Autodesk Fusion 360 part; units mm, degrees
(part 3 of 5)
  line L3 (45.4352, 19.4331, 2.5409) -> (44.7866, 20.9539, 2.7513) construction
  line L4 (44.7866, 20.9539, 2.7513) -> (44.0616, 22.4421, 2.9616) construction
  line L5 (44.0616, 22.4421, 2.9616) -> (43.2623, 23.8896, 3.172) construction
  line L6 (43.2623, 23.8896, 3.172) -> (39.2446, 31.1652, 4.2293) construction
  line L7 (39.2446, 31.1652, 4.2293) -> (33.358, 37.3986, 5.2866) construction
  line L8 (33.358, 37.3986, 5.2866) -> (26.324, 41.8256, 6.3439) construction
  line L9 (26.324, 41.8256, 6.3439) -> (19.2902, 46.2525, 7.4011) construction
  line L10 (19.2902, 46.2525, 7.4011) -> (11.1241, 48.8637, 8.4584) construction
  line L11 (11.1241, 48.8637, 8.4584) -> (2.8268, 49.3391, 9.5157) construction
  line L12 (2.8268, 49.3391, 9.5157) -> (-5.4704, 49.8145, 10.5729) construction
  line L13 (-5.4704, 49.8145, 10.5729) -> (-13.8811, 48.1531, 11.6302) construction
  line L14 (-13.8811, 48.1531, 11.6302) -> (-21.3743, 44.5587, 12.6874) construction
  line L15 (-21.3743, 44.5587, 12.6874) -> (-28.8674, 40.9643, 13.7447) construction
  line L16 (-28.8674, 40.9643, 13.7447) -> (-35.4271, 35.4447, 14.8019) construction
  line L17 (-35.4271, 35.4447, 14.8019) -> (-40.2493, 28.6763, 15.8591) construction
  line L18 (-40.2493, 28.6763, 15.8591) -> (-45.0715, 21.908, 16.9163) construction
  line L19 (-45.0715, 21.908, 16.9163) -> (-48.146, 13.9055, 17.9735) construction
  line L20 (-48.146, 13.9055, 17.9735) -> (-49.096, 5.6496, 19.0307) construction
  line L21 (-49.096, 5.6496, 19.0307) -> (-50.046, -2.606, 20.0879) construction
  line L22 (-50.046, -2.606, 20.0879) -> (-48.8696, -11.0975, 21.1451) construction
  line L23 (-48.8696, -11.0975, 21.1451) -> (-45.711, -18.784, 22.2022) construction
  line L24 (-45.711, -18.784, 22.2022) -> (-42.5525, -26.4703, 23.2594) construction
  line L25 (-42.5525, -26.4703, 23.2594) -> (-37.4186, -33.3353, 24.3165) construction
  line L26 (-37.4186, -33.3353, 24.3165) -> (-30.9385, -38.5376, 25.3737) construction
  line L27 (-30.9385, -38.5376, 25.3737) -> (-24.4586, -43.7398, 26.4308) construction
  line L28 (-24.4586, -43.7398, 26.4308) -> (-16.6463, -47.2683, 27.4879) construction
  line L29 (-16.6463, -47.2683, 27.4879) -> (-8.4592, -48.6906, 28.545) construction
  line L30 (-8.4592, -48.6906, 28.545) -> (-0.2722, -50.113, 29.6021) construction
  line L31 (-0.2722, -50.113, 29.6021) -> (8.2721, -49.4263, 30.6592) construction
  line L32 (8.2721, -49.4263, 30.6592) -> (16.1268, -46.7147, 31.7163) construction
  line L33 (16.1268, -46.7147, 31.7163) -> (23.9813, -44.0032, 32.7734) construction
  line L34 (23.9813, -44.0032, 32.7734) -> (31.1295, -39.2726, 33.8305) construction
  line L35 (31.1295, -39.2726, 33.8305) -> (36.6953, -33.1027, 34.8876) construction
  line L36 (36.6953, -33.1027, 34.8876) -> (42.261, -26.933, 35.9446) construction
  line L37 (42.261, -26.933, 35.9446) -> (46.2326, -19.3372, 37.0017) construction
  line L38 (46.2326, -19.3372, 37.0017) -> (48.1234, -11.246, 38.0587) construction
  line L39 (48.1234, -11.246, 38.0587) -> (50.0142, -3.155, 39.1157) construction
  line L40 (50.0142, -3.155, 39.1157) -> (49.8203, 5.4141, 40.1728) construction
  line L41 (49.8203, 5.4141, 40.1728) -> (47.5655, 13.4113, 41.2298) construction
  line L42 (47.5655, 13.4113, 41.2298) -> (45.3107, 21.4083, 42.2868) construction
  line L43 (45.3107, 21.4083, 42.2868) -> (40.9999, 28.8164, 43.3438) construction
  line L44 (40.9999, 28.8164, 43.3438) -> (35.1612, 34.7279, 44.4008) construction
  line L45 (35.1612, 34.7279, 44.4008) -> (29.3227, 40.6393, 45.4577) construction
  line L46 (29.3227, 40.6393, 45.4577) -> (21.9688, 45.0415, 46.5147) construction
  line L47 (21.9688, 45.0415, 46.5147) -> (14.0006, 47.3954, 47.5717) construction
  line L48 (14.0006, 47.3954, 47.5717) -> (6.0326, 49.7491, 48.6286) construction
  line L49 (6.0326, 49.7491, 48.6286) -> (-2.5328, 50.0495, 49.6856) construction
  line L50 (-2.5328, 50.0495, 49.6856) -> (-10.6461, 48.2597, 50.7425) construction
  line L51 (-10.6461, 48.2597, 50.7425) -> (-18.7593, 46.4699, 51.7995) construction
  line L52 (-18.7593, 46.4699, 51.7995) -> (-26.4031, 42.5939, 52.8564) construction
  line L53 (-26.4031, 42.5939, 52.8564) -> (-32.6413, 37.1064, 53.9133) construction
  line L54 (-32.6413, 37.1064, 53.9133) -> (-38.8792, 31.6191, 54.9702) construction
  line L55 (-38.8792, 31.6191, 54.9702) -> (-43.6983, 24.5321, 56.0271) construction
  line L56 (-43.6983, 24.5321, 56.0271) -> (-46.508, 16.7136, 57.084) construction
  line L57 (-46.508, 16.7136, 57.084) -> (-49.3176, 8.8953, 58.1409) construction
  line L58 (-49.3176, 8.8953, 58.1409) -> (-50.1121, 0.3622, 59.1978) construction
  line L59 (-50.1121, 0.3622, 59.1978) -> (-48.7941, -7.8404, 60.2546) construction
  line L60 (-48.7941, -7.8404, 60.2546) -> (-47.4761, -16.0429, 61.3115) construction
  line L61 (-47.4761, -16.0429, 61.3115) -> (-44.0485, -23.8973, 62.3684) construction
  line L62 (-44.0485, -23.8973, 62.3684) -> (-38.9312, -30.4418, 63.4252) construction
  line L63 (-38.9312, -30.4418, 63.4252) -> (-33.8139, -36.986, 64.482) construction
  line L64 (-33.8139, -36.986, 64.482) -> (-27.0179, -42.2064, 65.5389) construction
  line L65 (-27.0179, -42.2064, 65.5389) -> (-19.3756, -45.4634, 66.5957) construction
  line L66 (-19.3756, -45.4634, 66.5957) -> (-11.7334, -48.7204, 67.6525) construction
  line L67 (-11.7334, -48.7204, 67.6525) -> (-3.2612, -50.0071, 68.7093) construction
  line L68 (-3.2612, -50.0071, 68.7093) -> (5.0034, -49.1661, 69.7661) construction
  line L69 (5.0034, -49.1661, 69.7661) -> (13.2677, -48.3251, 70.8229) construction
  line L70 (13.2677, -48.3251, 70.8229) -> (21.3069, -45.3581, 71.8796) construction
  line L71 (21.3069, -45.3581, 71.8796) -> (28.1362, -40.6287, 72.9364) construction
  line L72 (28.1362, -40.6287, 72.9364) -> (34.9654, -35.8993, 73.9932) construction
  line L73 (34.9654, -35.8993, 73.9932) -> (40.5702, -29.4176, 75.0499) construction
  line L74 (40.5702, -29.4176, 75.0499) -> (44.2643, -21.9774, 76.1067) construction
  line L75 (44.2643, -21.9774, 76.1067) -> (47.9584, -14.5373, 77.1634) construction
  line L76 (47.9584, -14.5373, 77.1634) -> (49.7339, -6.1545, 78.2202) construction
  line L77 (49.7339, -6.1545, 78.2202) -> (49.3735, 2.1444, 79.2769) construction
  line L78 (49.3735, 2.1444, 79.2769) -> (49.013, 10.4431, 80.3336) construction
  line L79 (49.013, 10.4431, 80.3336) -> (46.5175, 18.6401, 81.3903) construction
  line L80 (46.5175, 18.6401, 81.3903) -> (42.1925, 25.7318, 82.447) construction
  line L81 (42.1925, 25.7318, 82.447) -> (37.8676, 32.8234, 83.5037) construction
  line L82 (37.8676, 32.8234, 83.5037) -> (31.7225, 38.7945, 84.5604) construction
  line L83 (31.7225, 38.7945, 84.5604) -> (24.5097, 42.914, 85.617) construction
  line L84 (24.5097, 42.914, 85.617) -> (17.2971, 47.0334, 86.6737) construction
  line L85 (17.2971, 47.0334, 86.6737) -> (9.0322, 49.2925, 87.7304) construction
  line L86 (9.0322, 49.2925, 87.7304) -> (0.7269, 49.4147, 88.787) construction
  line L87 (0.7269, 49.4147, 88.787) -> (-7.5781, 49.5368, 89.8437) construction
  line L88 (-7.5781, 49.5368, 89.8437) -> (-15.9057, 47.5219, 90.9003) construction
  line L89 (-15.9057, 47.5219, 90.9003) -> (-23.2363, 43.6166, 91.9569) construction
  line L90 (-23.2363, 43.6166, 91.9569) -> (-30.5667, 39.7114, 93.0135) construction
  line L91 (-30.5667, 39.7114, 93.0135) -> (-36.8845, 33.9243, 94.0701) construction
  line L92 (-36.8845, 33.9243, 94.0701) -> (-41.4161, 26.9637, 95.1268) construction
  line L93 (-41.4161, 26.9637, 95.1268) -> (-45.9477, 20.0033, 96.1833) construction
  line L94 (-45.9477, 20.0033, 96.1833) -> (-48.6835, 11.8843, 97.2399) construction
  line L95 (-48.6835, 11.8843, 97.2399) -> (-49.2886, 3.6009, 98.2965) construction
  line L96 (-49.2886, 3.6009, 98.2965) -> (-49.8938, -4.6824, 99.3531) construction
  line L97 (-49.8938, -4.6824, 99.3531) -> (-48.3671, -13.1126, 100.4096) construction
  line L98 (-48.3671, -13.1126, 100.4096) -> (-44.8954, -20.6576, 101.4662) construction
  line L99 (-44.8954, -20.6576, 101.4662) -> (-41.4239, -28.2024, 102.5227) construction
  line L100 (-41.4239, -28.2024, 102.5227) -> (-36.0148, -34.846, 103.5793) construction
  line L101 (-36.0148, -34.846, 103.5793) -> (-29.3305, -39.7751, 104.6358) construction
  line L102 (-29.3305, -39.7751, 104.6358) -> (-22.6463, -44.7041, 105.6923) construction
  line L103 (-22.6463, -44.7041, 105.6923) -> (-14.7012, -47.9081, 106.7488) construction
  line L104 (-14.7012, -47.9081, 106.7488) -> (-6.4676, -48.995, 107.8054) construction
  line L105 (-6.4676, -48.995, 107.8054) -> (1.7658, -50.0818, 108.8619) construction
  line L106 (1.7658, -50.0818, 108.8619) -> (10.27, -49.0493, 109.9183) construction
  line L107 (10.27, -49.0493, 109.9183) -> (18.0041, -46.0238, 110.9748) construction
  line L108 (18.0041, -46.0238, 110.9748) -> (25.738, -42.9983, 112.0313) construction
  line L109 (25.738, -42.9983, 112.0313) -> (32.6854, -37.9864, 113.0878) construction
  line L110 (32.6854, -37.9864, 113.0878) -> (37.9957, -31.6016, 114.1442) construction
  line L111 (37.9957, -31.6016, 114.1442) -> (43.306, -25.2168, 115.2007) construction
  line L112 (43.306, -25.2168, 115.2007) -> (46.9681, -17.4728, 116.2571) construction
  line L113 (46.9681, -17.4728, 116.2571) -> (48.5337, -9.3173, 117.3136) construction
  line L114 (48.5337, -9.3173, 117.3136) -> (50.0994, -1.1619, 118.37) construction
  line L115 (50.0994, -1.1619, 118.37) -> (49.5653, 7.3875, 119.4264) construction
  line L116 (49.5653, 7.3875, 119.4264) -> (46.997, 15.2846, 120.4828) construction
  line L117 (46.997, 15.2846, 120.4828) -> (44.4287, 23.1815, 121.5392) construction
  line L118 (44.4287, 23.1815, 121.5392) -> (39.8317, 30.4094, 122.5956) construction
  line L119 (39.8317, 30.4094, 122.5956) -> (33.7686, 36.0835, 123.652) construction
  line L120 (33.7686, 36.0835, 123.652) -> (27.7056, 41.7575, 124.7084) construction
  line L121 (27.7056, 41.7575, 124.7084) -> (20.1894, 45.8659, 125.7648) construction
  line L122 (20.1894, 45.8659, 125.7648) -> (12.14, 47.9057, 126.8211) construction
  line L123 (12.14, 47.9057, 126.8211) -> (4.0907, 49.9455, 127.8775) construction
  line L124 (4.0907, 49.9455, 127.8775) -> (-4.4747, 49.9126, 128.9338) construction
  line L125 (-4.4747, 49.9126, 128.9338) -> (-12.508, 47.8109, 129.9902) construction
  line L126 (-12.508, 47.8109, 129.9902) -> (-20.5412, 45.7093, 131.0465) construction
  line L127 (-20.5412, 45.7093, 131.0465) -> (-28.0252, 41.5436, 132.1029) construction
  line L128 (-28.0252, 41.5436, 132.1029) -> (-34.0443, 35.8235, 133.1592) construction
  line L129 (-34.0443, 35.8235, 133.1592) -> (-40.0632, 30.1035, 134.2155) construction
  line L130 (-40.0632, 30.1035, 134.2155) -> (-44.6044, 22.8414, 135.2718) construction
  line L131 (-44.6044, 22.8414, 135.2718) -> (-47.1122, 14.9259, 136.3281) construction
  line L132 (-47.1122, 14.9259, 136.3281) -> (-49.6199, 7.0105, 137.3844) construction
  line L133 (-49.6199, 7.0105, 137.3844) -> (-50.0889, -1.5416, 138.4407) construction
  line L134 (-50.0889, -1.5416, 138.4407) -> (-48.462, -9.6838, 139.4969) construction
  line L135 (-48.462, -9.6838, 139.4969) -> (-46.835, -17.8258, 140.5532) construction
  line L136 (-46.835, -17.8258, 140.5532) -> (-43.1155, -25.5407, 141.6095) construction
  line L137 (-43.1155, -25.5407, 141.6095) -> (-37.7587, -31.8844, 142.6657) construction
  line L138 (-37.7587, -31.8844, 142.6657) -> (-32.402, -38.2281, 143.7219) construction
  line L139 (-32.402, -38.2281, 143.7219) -> (-25.4193, -43.1872, 144.7782) construction
  line L140 (-25.4193, -43.1872, 144.7782) -> (-17.665, -46.155, 145.8344) construction
  line L141 (-17.665, -46.155, 145.8344) -> (-9.911, -49.1227, 146.8906) construction
  line L142 (-9.911, -49.1227, 146.8906) -> (-1.4018, -50.093, 147.9468) construction
  line L143 (-1.4018, -50.093, 147.9468) -> (6.8213, -48.947, 149.0031) construction
  line L144 (6.8213, -48.947, 149.0031) -> (15.0443, -47.801, 150.0592) construction
  line L145 (15.0443, -47.801, 150.0592) -> (22.9638, -44.5413, 151.1154) construction
  line L146 (22.9638, -44.5413, 151.1154) -> (29.6109, -39.5668, 152.1716) construction
  line L147 (29.6109, -39.5668, 152.1716) -> (36.2579, -34.5923, 153.2278) construction
  line L148 (36.2579, -34.5923, 153.2278) -> (41.6184, -27.9136, 154.284) construction
  line L149 (41.6184, -27.9136, 154.284) -> (45.0367, -20.3478, 155.3401) construction
  line L150 (45.0367, -20.3478, 155.3401) -> (48.4549, -12.782, 156.3963) construction
  line L151 (48.4549, -12.782, 156.3963) -> (49.9237, -4.3452, 157.4524) construction
  line L152 (49.9237, -4.3452, 157.4524) -> (49.2634, 3.9305, 158.5085) construction
  line L153 (49.2634, 3.9305, 158.5085) -> (48.6032, 12.2061, 159.5647) construction
  line L154 (48.6032, 12.2061, 159.5647) -> (45.8153, 20.3031, 160.6208) construction
  line L155 (45.8153, 20.3031, 160.6208) -> (41.2409, 27.231, 161.6769) construction
  line L156 (41.2409, 27.231, 161.6769) -> (36.6665, 34.1588, 162.733) construction
  line L157 (36.6665, 34.1588, 162.733) -> (30.3154, 39.9028, 163.7891) construction
  line L158 (30.3154, 39.9028, 163.7891) -> (22.9644, 43.7604, 164.8452) construction
  line L159 (22.9644, 43.7604, 164.8452) -> (15.6136, 47.6179, 165.9013) construction
  line L160 (15.6136, 47.6179, 165.9013) -> (7.2785, 49.581, 166.9574) construction
  line L161 (7.2785, 49.581, 166.9574) -> (-1.0213, 49.4094, 168.0134) construction
  line L162 (-1.0213, 49.4094, 168.0134) -> (-9.3208, 49.2379, 169.0695) construction
  line L163 (-9.3208, 49.2379, 169.0695) -> (-17.5675, 46.9322, 170.1255) construction
  line L164 (-17.5675, 46.9322, 170.1255) -> (-24.7525, 42.7744, 171.1816) construction
  line L165 (-24.7525, 42.7744, 171.1816) -> (-31.9374, 38.6166, 172.2376) construction
  line L166 (-31.9374, 38.6166, 172.2376) -> (-38.0455, 32.6157, 173.2936) construction
  line L167 (-38.0455, 32.6157, 173.2936) -> (-42.3297, 25.5055, 174.3497) construction
  line L168 (-42.3297, 25.5055, 174.3497) -> (-46.6139, 18.3954, 175.4057) construction
  line L169 (-46.6139, 18.3954, 175.4057) -> (-49.0651, 10.1912, 176.4617) construction
  line L170 (-49.0651, 10.1912, 176.4617) -> (-49.3836, 1.8964, 177.5177) construction
  line L171 (-49.3836, 1.8964, 177.5177) -> (-49.7021, -6.3984, 178.5737) construction
  line L172 (-49.7021, -6.3984, 178.5737) -> (-47.8874, -14.7662, 179.6297) construction
  line L173 (-47.8874, -14.7662, 179.6297) -> (-44.1613, -22.1837, 180.6857) construction
  line L174 (-44.1613, -22.1837, 180.6857) -> (-40.4353, -29.6011, 181.7416) construction
  line L175 (-40.4353, -29.6011, 181.7416) -> (-34.8059, -36.0525, 182.7976) construction
  line L176 (-34.8059, -36.0525, 182.7976) -> (-27.9617, -40.749, 183.8535) construction
  line L177 (-27.9617, -40.749, 183.8535) -> (-21.1176, -45.4454, 184.9095) construction
  line L178 (-21.1176, -45.4454, 184.9095) -> (-13.0731, -48.3769, 185.9654) construction
  line L179 (-13.0731, -48.3769, 185.9654) -> (-4.8121, -49.1852, 187.0214) construction
  line L180 (-4.8121, -49.1852, 187.0214) -> (3.4487, -49.9934, 188.0773) construction
  line L181 (3.4487, -49.9934, 188.0773) -> (11.9086, -48.6766, 189.1332) construction
  line L182 (11.9086, -48.6766, 189.1332) -> (19.5331, -45.396, 190.1891) construction
  line L183 (19.5331, -45.396, 190.1891) -> (27.1574, -42.1154, 191.245) construction
  line L184 (27.1574, -42.1154, 191.245) -> (33.9301, -36.8779, 192.3009) construction
  line L185 (33.9301, -36.8779, 192.3009) -> (39.023, -30.324, 193.3568) construction
  line L186 (39.023, -30.324, 193.3568) -> (44.1158, -23.7702, 194.4127) construction
  line L187 (44.1158, -23.7702, 194.4127) -> (47.5181, -15.9139, 195.4685) construction
  line L188 (47.5181, -15.9139, 195.4685) -> (48.814, -7.7157, 196.5244) construction
  line L189 (48.814, -7.7157, 196.5244) -> (50.1098, 0.4823, 197.5803) construction
  line L190 (50.1098, 0.4823, 197.5803) -> (49.2964, 9.0047, 198.6361) construction
  line L191 (49.2964, 9.0047, 198.6361) -> (46.4733, 16.8097, 199.692) construction
  line L192 (46.4733, 16.8097, 199.692) -> (43.6503, 24.6144, 200.7478) construction
  line L193 (43.6503, 24.6144, 200.7478) -> (38.8237, 31.685, 201.8036) construction
  line L194 (38.8237, 31.685, 201.8036) -> (32.5835, 37.1571, 202.8595) construction
  line L195 (32.5835, 37.1571, 202.8595) -> (26.3435, 42.6291, 203.9153) construction
  line L196 (26.3435, 42.6291, 203.9153) -> (18.7032, 46.4909, 204.9711) construction
  line L197 (18.7032, 46.4909, 204.9711) -> (10.5968, 48.2705, 206.0269) construction
  line L198 (10.5968, 48.2705, 206.0269) -> (2.4906, 50.0501, 207.0827) construction
  line L199 (2.4906, 50.0501, 207.0827) -> (-6.0645, 49.7437, 208.1385) construction
  line L200 (-6.0645, 49.7437, 208.1385) -> (-14.0227, 47.3888, 209.1942) construction
  line L201 (-14.0227, 47.3888, 209.1942) -> (-21.9807, 45.034, 210.25) construction
  line L202 (-21.9807, 45.034, 210.25) -> (-29.3248, 40.6358, 211.3058) construction
  line L203 (-29.3248, 40.6358, 211.3058) -> (-35.1573, 34.7318, 212.3615) construction
  line L204 (-35.1573, 34.7318, 212.3615) -> (-40.9897, 28.828, 213.4173) construction
  line L205 (-40.9897, 28.828, 213.4173) -> (-45.2981, 21.431, 214.473) construction
  line L206 (-45.2981, 21.431, 214.473) -> (-47.5559, 13.4451, 215.5287) construction
  line L207 (-47.5559, 13.4451, 215.5287) -> (-49.8137, 5.4594, 216.5845) construction
  line L208 (-49.8137, 5.4594, 216.5845) -> (-50.0161, -3.0982, 217.6402) construction
  line L209 (-50.0161, -3.0982, 217.6402) -> (-48.1384, -11.1818, 218.6959) construction
  line L210 (-48.1384, -11.1818, 218.6959) -> (-46.2608, -19.2651, 219.7516) construction
  line L211 (-46.2608, -19.2651, 219.7516) -> (-42.3071, -26.8572, 220.8073) construction
  line L212 (-42.3071, -26.8572, 220.8073) -> (-36.7607, -33.0301, 221.863) construction
  line L213 (-36.7607, -33.0301, 221.863) -> (-31.2145, -39.2028, 222.9187) construction
  line L214 (-31.2145, -39.2028, 222.9187) -> (-24.0873, -43.9432, 223.9744) construction
  line L215 (-24.0873, -43.9432, 223.9744) -> (-16.2504, -46.6719, 225.03) construction
  line L216 (-16.2504, -46.6719, 225.03) -> (-8.4136, -49.4005, 226.0857) construction
  line L217 (-8.4136, -49.4005, 226.0857) -> (0.1163, -50.1117, 227.1413) construction
  line L218 (0.1163, -50.1117, 227.1413) -> (8.2968, -48.7186, 228.197) construction
  line L219 (8.2968, -48.7186, 228.197) -> (16.477, -47.3255, 229.2526) construction
  line L220 (16.477, -47.3255, 229.2526) -> (24.2905, -43.8311, 230.3083) construction
  line L221 (24.2905, -43.8311, 230.3083) -> (30.7823, -38.6625, 231.3639) construction
  line L222 (30.7823, -38.6625, 231.3639) -> (37.2739, -33.4939, 232.4195) construction
  line L223 (37.2739, -33.4939, 232.4195) -> (42.4301, -26.6622, 233.4751) construction
  line L224 (42.4301, -26.6622, 233.4751) -> (45.6207, -19.0023, 234.5307) construction
  line L225 (45.6207, -19.0023, 234.5307) -> (48.8112, -11.3425, 235.5863) construction
  line L226 (48.8112, -11.3425, 235.5863) -> (50.0295, -2.8707, 236.6419) construction
  line L227 (50.0295, -2.8707, 236.6419) -> (49.1265, 5.3778, 237.6975) construction
  line L228 (49.1265, 5.3778, 237.6975) -> (48.2236, 13.6261, 238.7531) construction
  line L229 (48.2236, 13.6261, 238.7531) -> (45.2015, 21.6335, 239.8086) construction
  line L230 (45.2015, 21.6335, 239.8086) -> (40.4296, 28.4216, 240.8642) construction
  line L231 (40.4296, 28.4216, 240.8642) -> (35.6577, 35.2095, 241.9197) construction
  line L232 (35.6577, 35.2095, 241.9197) -> (29.1462, 40.7637, 242.9753) construction
  line L233 (29.1462, 40.7637, 242.9753) -> (21.6908, 44.4055, 244.0308) construction
  line L234 (21.6908, 44.4055, 244.0308) -> (14.2354, 48.0472, 245.0864) construction
  line L235 (14.2354, 48.0472, 245.0864) -> (5.852, 49.7688, 246.1419) construction
  line L236 (5.852, 49.7688, 246.1419) -> (-2.4351, 49.36, 247.1974) construction
  line L237 (-2.4351, 49.36, 247.1974) -> (-10.7221, 48.9511, 248.2529) construction
  line L238 (-10.7221, 48.9511, 248.2529) -> (-18.8952, 46.4128, 249.3084) construction
  line L239 (-18.8952, 46.4128, 249.3084) -> (-25.9558, 42.0551, 250.3639) construction
  line L240 (-25.9558, 42.0551, 250.3639) -> (-33.0162, 37.6976, 251.4194) construction
  line L241 (-33.0162, 37.6976, 251.4194) -> (-38.9492, 31.5299, 252.4749) construction
  line L242 (-38.9492, 31.5299, 252.4749) -> (-43.0298, 24.3059, 253.5304) construction
  line L243 (-43.0298, 24.3059, 253.5304) -> (-47.1103, 17.082, 254.5858) construction
  line L244 (-47.1103, 17.082, 254.5858) -> (-49.3298, 8.817, 255.6413) construction
  line L245 (-49.3298, 8.817, 255.6413) -> (-49.4173, 0.5207, 256.6968) construction
  line L246 (-49.4173, 0.5207, 256.6968) -> (-49.5047, -7.7753, 257.7522) construction
  line L247 (-49.5047, -7.7753, 257.7522) -> (-47.4599, -16.0851, 258.8076) construction
  line L248 (-47.4599, -16.0851, 258.8076) -> (-43.5326, -23.3933, 259.8631) construction
  line L249 (-43.5326, -23.3933, 259.8631) -> (-39.6055, -30.7013, 260.9185) construction
  line L250 (-39.6055, -30.7013, 260.9185) -> (-33.8043, -36.9923, 261.9739) construction
  line L251 (-33.8043, -36.9923, 261.9739) -> (-26.8379, -41.4977, 263.0293) construction
  line L252 (-26.8379, -41.4977, 263.0293) -> (-19.8716, -46.0031, 264.0847) construction
  line L253 (-19.8716, -46.0031, 264.0847) -> (-11.7549, -48.7133, 265.1401) construction
  line L254 (-11.7549, -48.7133, 265.1401) -> (-3.4792, -49.2974, 266.1955) construction
  line L255 (-3.4792, -49.2974, 266.1955) -> (4.7962, -49.8814, 267.2509) construction
  line L256 (4.7962, -49.8814, 267.2509) -> (13.213, -48.3381, 268.3063) construction
  line L257 (13.213, -48.3381, 268.3063) -> (20.7429, -44.8561, 269.3617) construction
  line L258 (20.7429, -44.8561, 269.3617) -> (28.2727, -41.3741, 270.417) construction
  line L259 (28.2727, -41.3741, 270.417) -> (34.8997, -35.9607, 271.4724) construction
  line L260 (34.8997, -35.9607, 271.4724) -> (39.8143, -29.2773, 272.5277) construction
  line L261 (39.8143, -29.2773, 272.5277) -> (44.7288, -22.594, 273.5831) construction
  line L262 (44.7288, -22.594, 273.5831) -> (47.9207, -14.6548, 274.6384) construction
  line L263 (47.9207, -14.6548, 274.6384) -> (49, -6.4296, 275.6937) construction
  line L264 (49, -6.4296, 275.6937) -> (50.0792, 1.7954, 276.749) construction
  line L265 (50.0792, 1.7954, 276.749) -> (49.0437, 10.2891, 277.8044) construction
  line L266 (49.0437, 10.2891, 277.8044) -> (46.0199, 18.0139, 278.8597) construction
  line L267 (46.0199, 18.0139, 278.8597) -> (42.9962, 25.7386, 279.915) construction
  line L268 (42.9962, 25.7386, 279.915) -> (37.9907, 32.6781, 280.9703) construction
  line L269 (37.9907, 32.6781, 280.9703) -> (31.6148, 37.9848, 282.0256) construction
  line L270 (31.6148, 37.9848, 282.0256) -> (25.2389, 43.2914, 283.0808) construction
  line L271 (25.2389, 43.2914, 283.0808) -> (17.5063, 46.954, 284.1361) construction
  line L272 (17.5063, 46.954, 284.1361) -> (9.3612, 48.5253, 285.1914) construction
  line L273 (9.3612, 48.5253, 285.1914) -> (1.2163, 50.0966, 286.2466) construction
  line L274 (1.2163, 50.0966, 286.2466) -> (-7.3237, 49.5733, 287.3019) construction
  line L275 (-7.3237, 49.5733, 287.3019) -> (-15.2158, 47.0193, 288.3571) construction
  line L276 (-15.2158, 47.0193, 288.3571) -> (-23.1077, 44.4654, 289.4124) construction
  line L277 (-23.1077, 44.4654, 289.4124) -> (-30.3351, 39.8864, 290.4676) construction
  line L278 (-30.3351, 39.8864, 290.4676) -> (-36.0152, 33.8414, 291.5228) construction
  line L279 (-36.0152, 33.8414, 291.5228) -> (-41.6952, 27.7965, 292.578) construction
  line L280 (-41.6952, 27.7965, 292.578) -> (-45.816, 20.2986, 293.6333) construction
  line L281 (-45.816, 20.2986, 293.6333) -> (-47.8743, 12.2633, 294.6885) construction
  line L282 (-47.8743, 12.2633, 294.6885) -> (-49.9325, 4.2281, 295.7437) construction
  line L283 (-49.9325, 4.2281, 295.7437) -> (-49.924, -4.3274, 296.7988) construction
  line L284 (-49.924, -4.3274, 296.7988) -> (-47.8498, -12.3584, 297.854) construction
  line L285 (-47.8498, -12.3584, 297.854) -> (-45.7756, -20.3893, 298.9092) construction
  line L286 (-45.7756, -20.3893, 298.9092) -> (-41.6402, -27.8788, 299.9644) construction
  line L287 (-41.6402, -27.8788, 299.9644) -> (-35.9486, -33.9122, 301.0195) construction
  line L288 (-35.9486, -33.9122, 301.0195) -> (-30.257, -39.9455, 302.0747) construction
  line L289 (-30.257, -39.9455, 302.0747) -> (-23.0213, -44.5101, 303.1298) construction
  line L290 (-23.0213, -44.5101, 303.1298) -> (-15.1251, -47.0486, 304.185) construction
  line L291 (-15.1251, -47.0486, 304.185) -> (-7.229, -49.587, 305.2401) construction
  line L292 (-7.229, -49.587, 305.2401) -> (1.311, -50.094, 306.2953) construction
  line L293 (1.311, -50.094, 306.2953) -> (9.452, -48.5077, 307.3504) construction
  line L294 (9.452, -48.5077, 307.3504) -> (17.5928, -46.9214, 308.4055) construction
  line L295 (17.5928, -46.9214, 308.4055) -> (25.3175, -43.2452, 309.4606) construction
  line L296 (25.3175, -43.2452, 309.4606) -> (31.6828, -37.9281, 310.5157) construction
  line L297 (31.6828, -37.9281, 310.5157) -> (38.048, -32.611, 311.5708) construction
  line L298 (38.048, -32.611, 311.5708) -> (43.0403, -25.6642, 312.6259) construction
  line L299 (43.0403, -25.6642, 312.6259) -> (46.0504, -17.9359, 313.681) construction
  line L300 (46.0504, -17.9359, 313.681) -> (49.0604, -10.2078, 314.736) construction
  line L301 (49.0604, -10.2078, 314.736) -> (50.0817, -1.7145, 315.7911) construction
  line L302 (50.0817, -1.7145, 315.7911) -> (48.9898, 6.5069, 316.8462) construction
  line L303 (48.9898, 6.5069, 316.8462) -> (47.8978, 14.7282, 317.9012) construction
  line L304 (47.8978, 14.7282, 317.9012) -> (44.6949, 22.6602, 318.9563) construction
  line L305 (44.6949, 22.6602, 318.9563) -> (39.7721, 29.3346, 320.0113) construction
  line L306 (39.7721, 29.3346, 320.0113) -> (34.8494, 36.0088, 321.0664) construction
  line L307 (34.8494, 36.0088, 321.0664) -> (28.2172, 41.4114, 322.1214) construction
  line L308 (28.2172, 41.4114, 322.1214) -> (20.6853, 44.8827, 323.1764) construction
  line L309 (20.6853, 44.8827, 323.1764) -> (13.1536, 48.3539, 324.2314) construction
  line L310 (13.1536, 48.3539, 324.2314) -> (4.7381, 49.8865, 325.2864) construction
  line L311 (4.7381, 49.8865, 325.2864) -> (-3.5338, 49.2935, 326.3414) construction
  line L312 (-3.5338, 49.2935, 326.3414) -> (-11.8056, 48.7005, 327.3964) construction
  line L313 (-11.8056, 48.7005, 327.3964) -> (-19.9163, 45.9832, 328.4514) construction
  line L314 (-19.9163, 45.9832, 328.4514) -> (-26.8757, 41.4733, 329.5064) construction
  line L315 (-26.8757, 41.4733, 329.5064) -> (-33.8351, 36.9634, 330.5614) construction
  line L316 (-33.8351, 36.9634, 330.5614) -> (-39.6286, 30.6706, 331.6163) construction
  line L317 (-39.6286, 30.6706, 331.6163) -> (-43.5489, 23.3629, 332.6713) construction
  line L318 (-43.5489, 23.3629, 332.6713) -> (-47.4692, 16.0554, 333.7263) construction
  line L319 (-47.4692, 16.0554, 333.7263) -> (-49.5082, 7.7486, 334.7812) construction
  line L320 (-49.5082, 7.7486, 334.7812) -> (-49.417, -0.5436, 335.8362) construction
  line L321 (-49.417, -0.5436, 335.8362) -> (-49.3258, -8.8356, 336.8911) construction
  line L322 (-49.3258, -8.8356, 336.8911) -> (-47.1047, -17.0954, 337.946) construction
  line L323 (-47.1047, -17.0954, 337.946) -> (-43.0247, -24.3148, 339.0009) construction
  line L324 (-43.0247, -24.3148, 339.0009) -> (-38.9448, -31.5341, 340.0558) construction
  line L325 (-38.9448, -31.5341, 340.0558) -> (-33.0148, -37.6978, 341.1108) construction
  line L326 (-33.0148, -37.6978, 341.1108) -> (-25.9585, -42.0534, 342.1657) construction
  line L327 (-25.9585, -42.0534, 342.1657) -> (-18.9024, -46.409, 343.2206) construction
  line L328 (-18.9024, -46.409, 343.2206) -> (-10.7348, -48.9475, 344.2754) construction
  line L329 (-10.7348, -48.9475, 344.2754) -> (-2.4529, -49.3591, 345.3303) construction
  line L330 (-2.4529, -49.3591, 345.3303) -> (5.829, -49.7706, 346.3852) construction
  line L331 (5.829, -49.7706, 346.3852) -> (14.2078, -48.0545, 347.4401) construction
  line L332 (14.2078, -48.0545, 347.4401) -> (21.6609, -44.4201, 348.4949) construction
  line L333 (21.6609, -44.4201, 348.4949) -> (29.1139, -40.7857, 349.5498) construction
  line L334 (29.1139, -40.7857, 349.5498) -> (35.6255, -35.2408, 350.6046) construction
  line L335 (35.6255, -35.2408, 350.6046) -> (40.401, -28.4622, 351.6595) construction
  line L336 (40.401, -28.4622, 351.6595) -> (45.1764, -21.6836, 352.7143) construction
  line L337 (45.1764, -21.6836, 352.7143) -> (48.2057, -13.6857, 353.7692) construction
  line L338 (48.2057, -13.6857, 353.7692) -> (49.1192, -5.4444, 354.824) construction
  line L339 (49.1192, -5.4444, 354.824) -> (50.0326, 2.7967, 355.8788) construction
  line L340 (50.0326, 2.7967, 355.8788) -> (48.8284, 11.2637, 356.9336) construction
  line L341 (48.8284, 11.2637, 356.9336) -> (45.6535, 18.9234, 357.9884) construction
  line L342 (45.6535, 18.9234, 357.9884) -> (42.4786, 26.5829, 359.0432) construction
  line L343 (42.4786, 26.5829, 359.0432) -> (37.3398, 33.4189, 360.098) construction
  line L344 (37.3398, 33.4189, 360.098) -> (30.8642, 38.5971, 361.1528) construction
  line L345 (30.8642, 38.5971, 361.1528) -> (24.3887, 43.7753, 362.2076) construction
  line L346 (24.3887, 43.7753, 362.2076) -> (16.5901, 47.2848, 363.2623) construction
  line L347 (16.5901, 47.2848, 363.2623) -> (8.42, 48.6974, 364.3171) construction
  line L348 (8.42, 48.6974, 364.3171) -> (0.2501, 50.11, 365.3719) construction
  line L349 (0.2501, 50.11, 365.3719) -> (-8.274, 49.4229, 366.4266) construction
  line L350 (-8.274, 49.4229, 366.4266) -> (-16.1121, 46.7198, 367.4814) construction
  line L351 (-16.1121, 46.7198, 367.4814) -> (-23.9501, 44.0167, 368.5361) construction
  line L352 (-23.9501, 44.0167, 368.5361) -> (-31.0856, 39.3035, 369.5908) construction
  line L353 (-31.0856, 39.3035, 369.5908) -> (-36.6479, 33.1552, 370.6456) construction
  line L354 (-36.6479, 33.1552, 370.6456) -> (-42.2101, 27.0071, 371.7003) construction
  line L355 (-42.2101, 27.0071, 371.7003) -> (-46.1875, 19.4369, 372.755) construction
  line L356 (-46.1875, 19.4369, 372.755) -> (-48.0946, 11.3684, 373.8097) construction
  line L357 (-48.0946, 11.3684, 373.8097) -> (-50.0018, 3.3001, 374.8644) construction
  line L358 (-50.0018, 3.3001, 374.8644) -> (-49.8349, -5.2495, 375.9191) construction
  line L359 (-49.8349, -5.2495, 375.9191) -> (-47.6142, -13.2373, 376.9738) construction
  line L360 (-47.6142, -13.2373, 376.9738) -> (-45.3936, -21.2249, 378.0285) construction
  line L361 (-45.3936, -21.2249, 378.0285) -> (-41.1239, -28.6337, 379.0831) construction
  line L362 (-41.1239, -28.6337, 379.0831) -> (-35.3263, -34.56, 380.1378) construction
  line L363 (-35.3263, -34.56, 380.1378) -> (-29.5287, -40.4861, 381.1925) construction
  line L364 (-29.5287, -40.4861, 381.1925) -> (-22.2154, -44.9171, 382.2471) construction
  line L365 (-22.2154, -44.9171, 382.2471) -> (-14.2786, -47.3123, 383.3018) construction
  line L366 (-14.2786, -47.3123, 383.3018) -> (-6.3419, -49.7076, 384.3564) construction
  line L367 (-6.3419, -49.7076, 384.3564) -> (2.2015, -50.0621, 385.4111) construction
  line L368 (2.2015, -50.0621, 385.4111) -> (10.3093, -48.3327, 386.4657) construction
  line L369 (10.3093, -48.3327, 386.4657) -> (18.417, -46.6034, 387.5203) construction
  line L370 (18.417, -46.6034, 387.5203) -> (26.072, -42.7938, 388.5749) construction
  line L371 (26.072, -42.7938, 388.5749) -> (32.3406, -37.3688, 389.6296) construction
  line L372 (32.3406, -37.3688, 389.6296) -> (38.609, -31.9438, 390.6842) construction
  line L373 (38.609, -31.9438, 390.6842) -> (43.4777, -24.9149, 391.7388) construction
  line L374 (43.4777, -24.9149, 391.7388) -> (46.3527, -17.1395, 392.7933) construction
  line L375 (46.3527, -17.1395, 392.7933) -> (49.2277, -9.3642, 393.8479) construction
  line L376 (49.2277, -9.3642, 393.8479) -> (50.1031, -0.8589, 394.9025) construction
  line L377 (50.1031, -0.8589, 394.9025) -> (48.872, 7.339, 395.9571) construction
  line L378 (48.872, 7.339, 395.9571) -> (47.641, 15.5367, 397.0117) construction
  line L379 (47.641, 15.5367, 397.0117) -> (44.3062, 23.4097, 398.0662) construction
  line L380 (44.3062, 23.4097, 398.0662) -> (39.2745, 29.9975, 399.1208) construction
  line L381 (39.2745, 29.9975, 399.1208) -> (34.2428, 36.5852, 400.1753) construction
  line L382 (34.2428, 36.5852, 400.1753) -> (27.5249, 41.874, 401.2299) construction
  line L383 (27.5249, 41.874, 401.2299) -> (19.9401, 45.2187, 402.2844) construction
  line L384 (19.9401, 45.2187, 402.2844) -> (12.3555, 48.5633, 403.3389) construction
  line L385 (12.3555, 48.5633, 403.3389) -> (3.9201, 49.9568, 404.3935) construction
  line L386 (3.9201, 49.9568, 404.3935) -> (-4.3373, 49.2293, 405.448) construction
  line L387 (-4.3373, 49.2293, 405.448) -> (-12.5945, 48.5018, 406.5025) construction
  line L388 (-12.5945, 48.5018, 406.5025) -> (-20.6562, 45.6549, 407.557) construction
  line L389 (-20.6562, 45.6549, 407.557) -> (-27.5391, 41.0358, 408.6115) construction
  line L390 (-27.5391, 41.0358, 408.6115) -> (-34.4219, 36.4167, 409.666) construction
  line L391 (-34.4219, 36.4167, 409.666) -> (-40.1114, 30.0353, 410.7205) construction
  line L392 (-40.1114, 30.0353, 410.7205) -> (-43.9137, 22.6698, 411.775) construction
  line L393 (-43.9137, 22.6698, 411.775) -> (-47.716, 15.3044, 412.8294) construction
  line L394 (-47.716, 15.3044, 412.8294) -> (-49.6231, 6.9705, 413.8839) construction
  line L395 (-49.6231, 6.9705, 413.8839) -> (-49.4025, -1.3154, 414.9384) construction
  line L396 (-49.4025, -1.3154, 414.9384) -> (-49.1819, -9.6012, 415.9928) construction
  line L397 (-49.1819, -9.6012, 415.9928) -> (-46.834, -17.8217, 417.0473) construction
  line L398 (-46.834, -17.8217, 417.0473) -> (-42.6454, -24.9742, 418.1017) construction
  line L399 (-42.6454, -24.9742, 418.1017) -> (-38.4567, -32.1266, 419.1561) construction
  line L400 (-38.4567, -32.1266, 419.1561) -> (-32.4362, -38.196, 420.2106) construction
  line L401 (-32.4362, -38.196, 420.2106) -> (-25.3179, -42.4422, 421.265) construction
  line L402 (-25.3179, -42.4422, 421.265) -> (-18.1997, -46.6884, 422.3194) construction
  line L403 (-18.1997, -46.6884, 422.3194) -> (-9.9988, -49.1025, 423.3738) construction
  line L404 (-9.9988, -49.1025, 423.3738) -> (-1.7153, -49.3902, 424.4282) construction
  line L405 (-1.7153, -49.3902, 424.4282) -> (6.568, -49.6779, 425.4826) construction
  line L406 (6.568, -49.6779, 425.4826) -> (14.9165, -47.8386, 426.537) construction
  line L407 (14.9165, -47.8386, 426.537) -> (22.312, -44.0966, 427.5914) construction
  line L408 (22.312, -44.0966, 427.5914) -> (29.7074, -40.3547, 428.6458) construction
  line L409 (29.7074, -40.3547, 428.6458) -> (36.1343, -34.7181, 429.7002) construction
  line L410 (36.1343, -34.7181, 429.7002) -> (40.809, -27.874, 430.7546) construction
  line L411 (40.809, -27.874, 430.7546) -> (45.4837, -21.0301, 431.8089) construction
  line L412 (45.4837, -21.0301, 431.8089) -> (48.3963, -12.9933, 432.8633) construction
  line L413 (48.3963, -12.9933, 432.8633) -> (49.1918, -4.7435, 433.9176) construction
  line L414 (49.1918, -4.7435, 433.9176) -> (49.9873, 3.5061, 434.972) construction
  line L415 (49.9873, 3.5061, 434.972) -> (48.6641, 11.9513, 436.0263) construction
  line L416 (48.6641, 11.9513, 436.0263) -> (45.3834, 19.5622, 437.0806) construction
  line L417 (45.3834, 19.5622, 437.0806) -> (42.1028, 27.173, 438.135) construction
  line L418 (42.1028, 27.173, 438.135) -> (36.8718, 33.9336, 439.1893) construction
  line L419 (36.8718, 33.9336, 439.1893) -> (30.3282, 39.0197, 440.2436) construction
  line L420 (30.3282, 39.0197, 440.2436) -> (23.7847, 44.1056, 441.2979) construction
  line L421 (23.7847, 44.1056, 441.2979) -> (15.9425, 47.5064, 442.3522) construction
  line L422 (15.9425, 47.5064, 442.3522) -> (7.7576, 48.8073, 443.4065) construction
  line L423 (7.7576, 48.8073, 443.4065) -> (-0.4271, 50.1082, 444.4608) construction
  line L424 (-0.4271, 50.1082, 444.4608) -> (-8.9372, 49.3066, 445.5151) construction
  line L425 (-8.9372, 49.3066, 445.5151) -> (-16.735, 46.5003, 446.5694) construction
  line L426 (-16.735, 46.5003, 446.5694) -> (-24.5327, 43.694, 447.6236) construction
  line L427 (-24.5327, 43.694, 447.6236) -> (-31.6018, 38.8888, 448.6779) construction
  line L428 (-31.6018, 38.8888, 448.6779) -> (-37.0804, 32.6708, 449.7322) construction
  line L429 (-37.0804, 32.6708, 449.7322) -> (-42.5589, 26.4528, 450.7864) construction
  line L430 (-42.5589, 26.4528, 450.7864) -> (-46.4355, 18.835, 451.8407) construction
  line L431 (-46.4355, 18.835, 451.8407) -> (-48.2375, 10.7461, 452.8949) construction
  line L432 (-48.2375, 10.7461, 452.8949) -> (-50.0395, 2.6574, 453.9492) construction
  line L433 (-50.0395, 2.6574, 453.9492) -> (-49.7632, -5.8854, 455.0034) construction
  line L434 (-49.7632, -5.8854, 455.0034) -> (-47.4423, -13.8408, 456.0576) construction
  line L435 (-47.4423, -13.8408, 456.0576) -> (-45.1214, -21.7961, 457.1118) construction
  line L436 (-45.1214, -21.7961, 457.1118) -> (-40.7609, -29.1472, 458.166) construction
  line L437 (-40.7609, -29.1472, 458.166) -> (-34.8923, -34.9981, 459.2203) construction
  line L438 (-34.8923, -34.9981, 459.2203) -> (-29.0238, -40.8488, 460.2745) construction
  line L439 (-29.0238, -40.8488, 460.2745) -> (-21.6597, -45.187, 461.3287) construction
  line L440 (-21.6597, -45.187, 461.3287) -> (-13.6976, -47.4838, 462.3829) construction
  line L441 (-13.6976, -47.4838, 462.3829) -> (-5.7356, -49.7806, 463.437) construction
  line L442 (-5.7356, -49.7806, 463.437) -> (2.8075, -50.0312, 464.4912) construction
  line L443 (2.8075, -50.0312, 464.4912) -> (10.8904, -48.2051, 465.5454) construction
  line L444 (10.8904, -48.2051, 465.5454) -> (18.9732, -46.3791, 466.5995) construction
  line L445 (18.9732, -46.3791, 466.5995) -> (26.5788, -42.4803, 467.6537) construction
  line L446 (26.5788, -42.4803, 467.6537) -> (32.78, -36.9839, 468.7079) construction
  line L447 (32.78, -36.9839, 468.7079) -> (38.9812, -31.4876, 469.762) construction
  line L448 (38.9812, -31.4876, 469.762) -> (43.765, -24.4054, 470.8162) construction
  line L449 (43.765, -24.4054, 470.8162) -> (46.5485, -16.6005, 471.8703) construction
  line L450 (46.5485, -16.6005, 471.8703) -> (49.3319, -8.7958, 472.9244) construction
  line L451 (49.3319, -8.7958, 472.9244) -> (50.109, -0.2849, 473.9785) construction
  line L452 (50.109, -0.2849, 473.9785) -> (48.7853, 7.8949, 475.0327) construction
  line L453 (48.7853, 7.8949, 475.0327) -> (47.4616, 16.0746, 476.0868) construction
  line L454 (47.4616, 16.0746, 476.0868) -> (44.0398, 23.9058, 477.1409) construction
  line L455 (44.0398, 23.9058, 477.1409) -> (38.937, 30.4343, 478.195) construction
  line L456 (38.937, 30.4343, 478.195) -> (33.8343, 36.9626, 479.2491) construction
  line L457 (33.8343, 36.9626, 479.2491) -> (27.0614, 42.1743, 480.3032) construction
  line L458 (27.0614, 42.1743, 480.3032) -> (19.4437, 45.4343, 481.3573) construction
  line L459 (19.4437, 45.4343, 481.3573) -> (11.8261, 48.6943, 482.4113) construction
  line L460 (11.8261, 48.6943, 482.4113) -> (3.3799, 49.9957, 483.4654) construction
  line L461 (3.3799, 49.9957, 483.4654) -> (-4.8656, 49.1799, 484.5195) construction
  line L462 (-4.8656, 49.1799, 484.5195) -> (-13.111, 48.3641, 485.5735) construction
  line L463 (-13.111, 48.3641, 485.5735) -> (-21.1384, 45.433, 486.6276) construction
  line L464 (-21.1384, 45.433, 486.6276) -> (-27.9694, 40.7437, 487.6816) construction
  line L465 (-27.9694, 40.7437, 487.6816) -> (-34.8003, 36.0545, 488.7357) construction
  line L466 (-34.8003, 36.0545, 488.7357) -> (-40.4205, 29.6171, 489.7897) construction
  line L467 (-40.4205, 29.6171, 489.7897) -> (-44.1451, 22.2159, 490.8438) construction
  line L468 (-44.1451, 22.2159, 490.8438) -> (-47.8696, 14.8149, 491.8978) construction
  line L469 (-47.8696, 14.8149, 491.8978) -> (-49.6908, 6.4658, 492.9518) construction
  line L470 (-49.6908, 6.4658, 492.9518) -> (-49.3867, -1.814, 494.0058) construction
  line L471 (-49.3867, -1.814, 494.0058) -> (-49.0826, -10.0937, 495.0598) construction
  line L472 (-49.0826, -10.0937, 495.0598) -> (-46.6539, -18.2866, 496.1138) construction
  line L473 (-46.6539, -18.2866, 496.1138) -> (-42.3965, -25.3944, 497.1678) construction
  line L474 (-42.3965, -25.3944, 497.1678) -> (-38.1392, -32.502, 498.2218) construction
  line L475 (-38.1392, -32.502, 498.2218) -> (-32.0623, -38.5096, 499.2758) construction
  line L476 (-32.0623, -38.5096, 499.2758) -> (-24.9063, -42.685, 500.3298) construction
  line L477 (-24.9063, -42.685, 500.3298) -> (-17.7504, -46.8604, 501.3838) construction
  line L478 (-17.7504, -46.8604, 501.3838) -> (-9.5305, -49.195, 502.4377) construction
  line L479 (-9.5305, -49.195, 502.4377) -> (-1.2482, -49.4042, 503.4917) construction
  line L480 (-1.2482, -49.4042, 503.4917) -> (7.034, -49.6135, 504.5457) construction
  line L481 (7.034, -49.6135, 504.5457) -> (15.3612, -47.697, 505.5996) construction
  line L482 (15.3612, -47.697, 505.5996) -> (22.7187, -43.8884, 506.6536) construction
  line L483 (22.7187, -43.8884, 506.6536) -> (30.0762, -40.0799, 507.7075) construction
  line L484 (30.0762, -40.0799, 507.7075) -> (36.4484, -34.3873, 508.7614) construction
  line L485 (36.4484, -34.3873, 508.7614) -> (41.0592, -27.5041, 509.8154) construction
  line L486 (41.0592, -27.5041, 509.8154) -> (45.6699, -20.6211, 510.8693) construction
  line L487 (45.6699, -20.6211, 510.8693) -> (48.5094, -12.5622, 511.9232) construction
  line L488 (48.5094, -12.5622, 511.9232) -> (49.2318, -4.3092, 512.9771) construction
  line L489 (49.2318, -4.3092, 512.9771) -> (49.9541, 3.9437, 514.031) construction
  line L490 (49.9541, 3.9437, 514.031) -> (48.5579, 12.3733, 515.0849) construction
  line L491 (48.5579, 12.3733, 515.0849) -> (45.2132, 19.9525, 516.1388) construction
  line L492 (45.2132, 19.9525, 516.1388) -> (41.8685, 27.5317, 517.1927) construction
  line L493 (41.8685, 27.5317, 517.1927) -> (36.5825, 34.2445, 518.2466) construction
  line L494 (36.5825, 34.2445, 518.2466) -> (29.9991, 39.2733, 519.3005) construction
  line L495 (29.9991, 39.2733, 519.3005) -> (23.4158, 44.302, 520.3543) construction
  line L496 (23.4158, 44.302, 520.3543) -> (15.549, 47.636, 521.4082) construction
  line L497 (15.549, 47.636, 521.4082) -> (7.3571, 48.8693, 522.4621) construction
  line L498 (7.3571, 48.8693, 522.4621) -> (-0.8346, 50.1025, 523.5159) construction
  line L499 (-0.8346, 50.1025, 523.5159) -> (-9.3342, 49.2325, 524.5698) construction
  line L500 (-9.3342, 49.2325, 524.5698) -> (-17.1061, 46.365, 525.6236) construction
  line L501 (-17.1061, 46.365, 525.6236) -> (-24.878, 43.4977, 526.6775) construction
  line L502 (-24.878, 43.4977, 526.6775) -> (-31.9058, 38.6391, 527.7313) construction
  line L503 (-31.9058, 38.6391, 527.7313) -> (-37.3337, 32.3811, 528.7851) construction
  line L504 (-37.3337, 32.3811, 528.7851) -> (-42.7614, 26.1232, 529.8389) construction
  line L505 (-42.7614, 26.1232, 529.8389) -> (-46.5776, 18.4792, 530.8928) construction
  line L506 (-46.5776, 18.4792, 530.8928) -> (-48.3176, 10.3802, 531.9466) construction
  line L507 (-48.3176, 10.3802, 531.9466) -> (-50.0575, 2.2813, 533.0004) construction
  line L508 (-50.0575, 2.2813, 533.0004) -> (-49.7174, -6.2555, 534.0542) construction
  line L509 (-49.7174, -6.2555, 534.0542) -> (-47.3389, -14.1903, 535.108) construction
  line L510 (-47.3389, -14.1903, 535.108) -> (-44.9604, -22.125, 536.1618) construction
  line L511 (-44.9604, -22.125, 536.1618) -> (-40.5485, -29.441, 537.2156) construction
  line L512 (-40.5485, -29.441, 537.2156) -> (-34.6405, -35.2473, 538.2693) construction
  line L513 (-34.6405, -35.2473, 538.2693) -> (-28.7326, -41.0535, 539.3231) construction
  line L514 (-28.7326, -41.0535, 539.3231) -> (-21.3412, -45.3377, 540.3769) construction
  line L515 (-21.3412, -45.3377, 540.3769) -> (-13.3665, -47.5781, 541.4306) construction
  line L516 (-13.3665, -47.5781, 541.4306) -> (-5.392, -49.8184, 542.4844) construction
  line L517 (-5.392, -49.8184, 542.4844) -> (3.149, -50.0103, 543.5381) construction
  line L518 (3.149, -50.0103, 543.5381) -> (11.2161, -48.1304, 544.5919) construction
  line L519 (11.2161, -48.1304, 544.5919) -> (19.2831, -46.2505, 545.6456) construction
  line L520 (19.2831, -46.2505, 545.6456) -> (26.8593, -42.3028, 546.6994) construction
  line L521 (26.8593, -42.3028, 546.6994) -> (33.0218, -36.7681, 547.7531) construction
  line L522 (33.0218, -36.7681, 547.7531) -> (39.1843, -31.2335, 548.8068) construction
  line L523 (39.1843, -31.2335, 548.8068) -> (43.9203, -24.1236, 549.8605) construction
  line L524 (43.9203, -24.1236, 549.8605) -> (46.653, -16.3044, 550.9143) construction
  line L525 (46.653, -16.3044, 550.9143) -> (49.3857, -8.4852, 551.968) construction
  line L526 (49.3857, -8.4852, 551.968) -> (50.1093, 0.0268, 553.0217) construction
  line L527 (50.1093, 0.0268, 553.0217) -> (48.7358, 8.195, 554.0754) construction
  line L528 (48.7358, 8.195, 554.0754) -> (47.3623, 16.3631, 555.129) construction
  line L529 (47.3623, 16.3631, 555.129) -> (43.8947, 24.1702, 556.1827) construction
  line L530 (43.8947, 24.1702, 556.1827) -> (38.7552, 30.6655, 557.2364) construction
  line L531 (38.7552, 30.6655, 557.2364) -> (33.6157, 37.1607, 558.2901) construction
  line L532 (33.6157, 37.1607, 558.2901) -> (26.8153, 42.3306, 559.3438) construction
  line L533 (26.8153, 42.3306, 559.3438) -> (19.182, 45.5454, 560.3974) construction
  line L534 (19.182, 45.5454, 560.3974) -> (11.5489, 48.7602, 561.4511) construction
  line L535 (11.5489, 48.7602, 561.4511) -> (3.099, 50.0133, 562.5047) construction
  line L536 (3.099, 50.0133, 562.5047) -> (-5.1386, 49.1521, 563.5584) construction
  line L537 (-5.1386, 49.1521, 563.5584) -> (-13.3761, 48.2909, 564.612) construction
  line L538 (-13.3761, 48.2909, 564.612) -> (-21.3839, 45.3173, 565.6657) construction
  line L539 (-21.3839, 45.3173, 565.6657) -> (-28.1871, 40.5934, 566.7193) construction
  line L540 (-28.1871, 40.5934, 566.7193) -> (-34.9901, 35.8696, 567.7729) construction
  line L541 (-34.9901, 35.8696, 567.7729) -> (-40.574, 29.4054, 568.8265) construction
  line L542 (-40.574, 29.4054, 568.8265) -> (-44.259, 21.9881, 569.8802) construction
  line L543 (-44.259, 21.9881, 569.8802) -> (-47.9439, 14.5709, 570.9338) construction
  line L544 (-47.9439, 14.5709, 570.9338) -> (-49.7221, 6.2162, 571.9874) construction
  line L545 (-49.7221, 6.2162, 571.9874) -> (-49.3771, -2.0588, 573.041) construction
  line L546 (-49.3771, -2.0588, 573.041) -> (-49.0321, -10.3336, 574.0946) construction
  line L547 (-49.0321, -10.3336, 574.0946) -> (-46.5646, -18.5112, 575.1482) construction
  line L548 (-46.5646, -18.5112, 575.1482) -> (-42.2752, -25.5958, 576.2017) construction
  line L549 (-42.2752, -25.5958, 576.2017) -> (-37.9858, -32.6803, 577.2553) construction
  line L550 (-37.9858, -32.6803, 577.2553) -> (-31.8835, -38.657, 578.3089) construction
  line L551 (-31.8835, -38.657, 578.3089) -> (-24.7113, -42.7982, 579.3625) construction
  line L552 (-24.7113, -42.7982, 579.3625) -> (-17.5393, -46.9393, 580.416) construction
  line L553 (-17.5393, -46.9393, 580.416) -> (-9.3124, -49.2362, 581.4696) construction
  line L554 (-9.3124, -49.2362, 581.4696) -> (-1.0325, -49.4092, 582.5231) construction
  line L555 (-1.0325, -49.4092, 582.5231) -> (7.2473, -49.5822, 583.5767) construction
  line L556 (7.2473, -49.5822, 583.5767) -> (15.5628, -47.6311, 584.6302) construction
  line L557 (15.5628, -47.6311, 584.6302) -> (22.9015, -43.7933, 585.6838) construction
  line L558 (22.9015, -43.7933, 585.6838) -> (30.2402, -39.9556, 586.7373) construction
  line L559 (30.2402, -39.9556, 586.7373) -> (36.5866, -34.2395, 587.7908) construction
  line L560 (36.5866, -34.2395, 587.7908) -> (41.1682, -27.3407, 588.8443) construction
  line L561 (41.1682, -27.3407, 588.8443) -> (45.7497, -20.4421, 589.8979) construction
  line L562 (45.7497, -20.4421, 589.8979) -> (48.5568, -12.3755, 590.9514) construction
  line L563 (48.5568, -12.3755, 590.9514) -> (49.2477, -4.123, 592.0049) construction
  line L564 (49.2477, -4.123, 592.0049) -> (49.9386, 4.1294, 593.0584) construction
  line L565 (49.9386, 4.1294, 593.0584) -> (48.5119, 12.5503, 594.1119) construction
  line L566 (48.5119, 12.5503, 594.1119) -> (45.1413, 20.1146, 595.1654) construction
  line L567 (45.1413, 20.1146, 595.1654) -> (41.7708, 27.6787, 596.2188) construction
  line L568 (41.7708, 27.6787, 596.2188) -> (36.4636, 34.3704, 597.2723) construction
  line L569 (36.4636, 34.3704, 597.2723) -> (29.8657, 39.3749, 598.3258) construction
  line L570 (29.8657, 39.3749, 598.3258) -> (23.2678, 44.3793, 599.3793) construction
  line L571 (23.2678, 44.3793, 599.3793) -> (15.3933, 47.686, 600.4327) construction
  line L572 (15.3933, 47.686, 600.4327) -> (7.2007, 48.8926, 601.4862) construction
  line L573 (7.2007, 48.8926, 601.4862) -> (-0.9918, 50.0992, 602.5396) construction
  line L574 (-0.9918, 50.0992, 602.5396) -> (-9.4852, 49.2031, 603.5931) construction
  line L575 (-9.4852, 49.2031, 603.5931) -> (-17.2455, 46.3134, 604.6465) construction
  line L576 (-17.2455, 46.3134, 604.6465) -> (-25.0058, 43.4237, 605.7) construction
  line L577 (-25.0058, 43.4237, 605.7) -> (-32.0166, 38.5466, 606.7534) construction
  line L578 (-32.0166, 38.5466, 606.7534) -> (-37.4247, 32.2758, 607.8068) construction
  line L579 (-37.4247, 32.2758, 607.8068) -> (-42.8328, 26.005, 608.8603) construction
  line L580 (-42.8328, 26.005, 608.8603) -> (-46.6267, 18.3537, 609.9137) construction